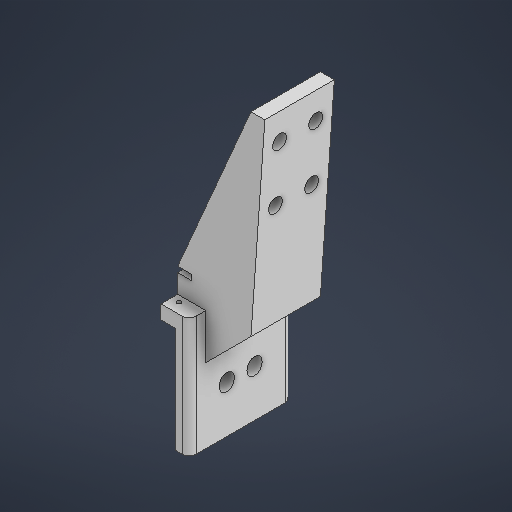
# Autodesk Inventor part: Camera_Bracket
Saved by Autodesk Inventor 2026 (Build 300175000, 175)
## iProperties
Created: 2025-04-19
Part Number: Camera_Bracket
Material: Generic
Document SubType Name: Modeling
Designer: Charl
Density: 1 g/cm^3
Appearance: Default
Author: Charl
Autodesk Inventor part; units mm, degrees
sketch "Sketch1" plane through (0, 0, 0) normal (0, 1, 0) x (-1, 0, 0)
  line L0 (-5.5, -37) -> (5.5, -37)
  line L1 (5.5, -37) -> (5.5, 37)
  line L2 (5.5, 37) -> (-5.5, 37)
  line L3 (-5.5, 37) -> (-5.5, -37)
  line L4 (-5.5, -37) -> (5.5, 37) construction
  line L5 (5.5, -37) -> (-5.5, 37) construction
  line L6 (-5.5, -25) -> (5.5, -25)
  line L7 (5.5, -25) -> (5.5, 25)
  line L8 (5.5, 25) -> (-5.5, 25)
  line L9 (-5.5, 25) -> (-5.5, -25)
  line L10 (-5.5, -25) -> (5.5, 25) construction
  line L11 (5.5, -25) -> (-5.5, 25) construction
  circle A0 centre (0, 29.5) radius 1.5
  circle A1 centre (0, -29.5) radius 1.5
  point P0 (0, 0)
  point P1 (0, -37)
  dimension "d0" = 74
  dimension "d1" = 11
  dimension "d2" = 11
  dimension "d3" = 50
  dimension "d4" = 3
  dimension "d5" = 7.5
  dimension "d6" = 3
  dimension "d7" = 7.5
  constraints: 24 end point, 5 midpoint, 4 parallel, 2 centre point, 2 horizontal, 2 perpendicular
  measures "d0" distance of L0.end L1.end
  measures "d1" distance of L1.end L2.end
  measures "d2" distance of L8.end L7.end
  measures "d3" distance of L7.end L6.end
  measures "d4" diameter of A0
  measures "d5" distance from line of A0.centre L2
  measures "d6" diameter of A1
  measures "d7" distance of point (0, -37) A1.centre
extrude "Extrusion1" add sketch "Sketch1" along normal blind 10
sketch "Sketch2" plane through (0, 10, 0) normal (0, 1, 0) x (1, 0, 0)
  line L0 (5.5, 37) -> (-5.5, 37) projected
  line L1 (4.8, 37) -> (14.8, 37)
  line L2 (14.8, 37) -> (14.8, -37)
  line L3 (14.8, -37) -> (4.8, -37)
  line L4 (4.8, -37) -> (4.8, 37)
  line L5 (5.5, -37) -> (5.5, 37) projected
  point P0 (0, 0)
  dimension "d10" = 74
  dimension "d11" = 0.7
  dimension "d12" = 10
  constraints: 8 end point, 2 parallel, 1 horizontal, 1 perpendicular, 1 point on line
  measures "d10" distance of L1.end L2.end
  measures "d11" distance between parallel lines of L5 L4
  measures "d12" distance of L1.start L1.end
extrude "Extrusion2" add sketch "Sketch2" against normal blind 86
ref_plane "Work Plane1" through (-5.5, 0, 0) normal (0, 0, 1) x (1, 0, 0)
sketch "Sketch3" plane through (-5.5, 0, 0) normal (0, 0, 1) x (1, 0, 0)
  line L0 (20.3, 10) -> (0, 10) projected
  line L1 (0, 10) -> (0, 27.494)
  line L2 (0, 27.494) -> (0.055, 27.494)
  line L3 (20.3, 10) -> (20.3, -76) projected
  line L4 (20.3, 10) -> (20.3, -22.405)
  line L5 (20.3, 10) -> (52.705, 10) construction
  line L6 (20.3, -22.405) -> (52.705, 10)
  line L7 (20.3, -22.405) -> (66.1276, -22.405) construction
  line L8 (52.705, 10) -> (52.705, 310)
  line L9 (52.705, 10) -> (352.705, 10) construction
  line L10 (0.055, 27.494) -> (10.055, 27.494) construction
  line L11 (52.705, 101.8003) -> (42.705, 101.8003) construction
  line L12 (42.705, 101.8003) -> (42.705, 219.1463) construction
  line L13 (42.705, 101.8003) -> (160.051, 101.8003) construction
  line L14 (0.055, 27.494) -> (42.705, 126.7645)
  line L15 (42.705, 126.7645) -> (52.705, 126.7645)
  point P0 (5.5, 0)
  dimension "d15" = 17.494
  dimension "d18" = 32.405
  dimension "d19" = 90
  dimension "d20" = 45
  dimension "d22" = 90
  dimension "d23" = 10
  dimension "d25" = 10
  dimension "d27" = 90
  dimension "d79" = 66.75
  constraints: 28 end point, 6 horizontal, 4 equal length, 3 point on line, 2 vertical, 1 collinear, 1 perpendicular
  measures "d15" distance of L0.end L1.end
  measures "d18" distance of L0.start L4.end
  measures "d19" angle of L4 L5
  measures "d20" angle of L7 L6
  measures "d22" angle of L9 L8
  measures "d23" distance of L2.end L10.end
  measures "d25" distance of L11.start L11.end
  measures "d27" angle of L13 L12
  measures "d79" angle of L10 L14
extrude "Extrusion3" add sketch "Sketch3" along normal mid plane 50
ref_plane "Work Plane2" through (-5.5, 27.494, 0) normal (-0.3947, -0.9188, 0) x (0, 0, 1)
sketch "Sketch4" plane through (-5.5, 0, 25) normal (0, 0, 1) x (1, 0, 0)
  line L0 (0, 0) -> (0, 10) construction
  line L1 (0, 10) -> (0, 23.494) construction
  line L2 (0, 23.494) -> (10, 23.494)
  line L3 (10, 23.494) -> (10, 27.494)
  line L4 (10, 27.494) -> (0, 27.494)
  line L5 (0, 27.494) -> (0, 23.494)
  point P0 (5.5, 0)
  dimension "d31" = 13.494
  dimension "d32" = 10
  dimension "d33" = 4
  constraints: 10 end point, 2 parallel, 1 horizontal, 1 perpendicular
  measures "d31" distance of L0.end L1.end
  measures "d32" distance of L4.end L3.end
  measures "d33" distance of L3.end L2.end
extrude "Extrusion4" cut sketch "Sketch4" against normal blind 269.75
sketch "Sketch5" plane through (-5.5, 27.494, 0) normal (-0.3947, -0.9188, 0) x (0, 0, 1)
  circle A0 centre (0, 14.9495) radius 25
  line L0 (-25, -0.0505) -> (25, -0.0505) projected
  point P0 (0, -15.9064)
  dimension "d36" = 50
  dimension "d37" = 15
  constraints: 1 centre point
  measures "d36" diameter of A0
  measures "d37" distance from line of L0 A0.centre
ref_plane "Work Plane3" through (37.205, 87.7645, 25) normal (0, 1, 0) x (1, 0, 0)
extrude "Extrusion5" cut sketch "Sketch5" along normal blind 54.3375 and the other way blind 67.371
ref_plane "Work Plane5" through (10.2593, -73.9067, 37) normal (-0.9081, 0.4187, 0) x (0, 0, 1)
ref_plane "Work Plane4" through (14.8, -76, 37) normal (-0.9081, 0.4187, 0) x (0, 0, 1)
sketch "Sketch6" plane through (10.2593, -73.9067, 37) normal (-0.9081, 0.4187, 0) x (0, 0, 1)
  line L0 (-74, 0) -> (0, 0) projected
  circle A0 centre (-37, 54.5) radius 5.5
  circle A1 centre (-37, 54.5) radius 2
  line L1 (-37, -200) -> (-37, 49)
  line L2 (-37, 60) -> (-37, 200)
  circle A2 centre (-47, 30.8) radius 5.5
  circle A3 centre (-47, 30.8) radius 2
  circle A4 centre (-27, 30.8) radius 5.5
  circle A5 centre (-27, 30.8) radius 2
  point P0 (-37, 62.8227)
  point P1 (-37, 0)
  dimension "d43" = 400
  dimension "d44" = 11
  dimension "d45" = 4
  dimension "d46" = 11
  dimension "d47" = 4
  dimension "d48" = 54.5
  dimension "d49" = 23.7
  dimension "d91" = 10
  constraints: 6 centre point, 4 end point, 3 coincident, 2 point on circle, 2 point on line, 2 symmetric about line, 2 vertical, 1 midpoint, 2 other
  measures "d43" distance of L1.start L2.end
  measures "d44" diameter of A0
  measures "d45" diameter of A1
  measures "d46" diameter of A2
  measures "d47" diameter of A3
  measures "d48" distance from line of L0 A0.centre
  measures "d49" vertical distance of A2.centre A0.centre
  measures "d91" distance from line of L1 A2.centre
extrude "Extrusion6" cut sketch "Sketch6" along normal blind 15 contours A0 | A1 | A2 | A3 | A4 | A5
extrude "Extrusion7" cut sketch "Sketch6" along normal blind 25.925 contours A0 | A1
extrude "Extrusion8" cut sketch "Sketch6" along normal blind 34.505 contours A1 | A3 | A5
ref_plane "Work Plane6" through (69.3627, 112.9485, -25) normal (-0.9188, 0.3947, 0) x (0, 0, 1)
sketch "Sketch7" plane through (69.3627, 112.9485, -25) normal (-0.9188, 0.3947, 0) x (0, 0, 1)
  line L0 (0, 0) -> (50, 0) projected
  line L1 (25, 150) -> (25, -150)
  line L2 (25, 150) -> (325, 150) construction
  line L3 (38, 10) -> (12, 10) construction
  line L4 (12, 10) -> (12, -29) construction
  line L5 (12, -29) -> (38, -29) construction
  line L6 (38, -29) -> (38, 10) construction
  circle A0 centre (38, 10) radius 2
  circle A1 centre (38, 10) radius 5
  circle A2 centre (38, -29) radius 2
  circle A3 centre (38, -29) radius 5
  circle A4 centre (12, 10) radius 2
  circle A5 centre (12, 10) radius 5
  circle A6 centre (12, -29) radius 2
  circle A7 centre (12, -29) radius 5
  line L7 (0, 3.9474) -> (50, 3.9474) projected
  point P0 (25, -131.1566)
  point P1 (25, 0)
  dimension "d57" = 300
  dimension "d58" = 90
  dimension "d63" = 26
  dimension "d64" = 39
  dimension "d67" = 4
  dimension "d68" = 10
  dimension "d69" = 10
  dimension "d70" = 4
  dimension "d78" = 13
  dimension "d85" = 10
  constraints: 12 end point, 8 centre point, 6 coincident, 4 symmetric about line, 2 horizontal, 2 midpoint, 2 parallel, 2 perpendicular, 1 vertical, 4 other
  measures "d57" distance of L1.start L1.end
  measures "d58" angle of L1 L2
  measures "d63" distance of L5.end L4.end
  measures "d64" distance of L4.end L3.end
  measures "d67" diameter of A0
  measures "d68" diameter of A1
  measures "d69" diameter of A3
  measures "d70" diameter of A2
  measures "d78" distance between parallel lines of L1 L6
  measures "d85" distance between parallel lines of L0 L3
fillet "Fillet1" radius 5 2 edges at (14.8, -33, 37) (14.8, -33, -37)
sketch "Sketch8" plane through (-5.5, 0, -25) normal (0, 0, -1) x (-1, 0, 0)
  line L0 (-52.705, 126.7645) -> (-42.705, 126.7645) construction
  line L1 (-42.705, 126.7645) -> (-52.705, 126.7645) construction
  line L2 (-52.705, 10) -> (-52.705, 126.7645) projected
  line L3 (-0.055, 27.494) -> (-42.705, 126.7645) projected
  line L4 (-42.705, 126.7645) -> (-52.705, 150.0402)
  line L5 (-52.705, 126.7645) -> (-42.705, 126.7645)
  line L6 (-52.705, 150.0402) -> (-62.705, 150.0402)
  line L7 (-62.705, 150.0402) -> (-52.705, 10)
  point P0 (-5.5, 0)
  dimension "d80" = 66.75
  dimension "d88" = 10
  constraints: 10 end point, 2 horizontal, 1 collinear, 1 point on line
  measures "d80" angle of L0 L4
  measures "d88" distance of L6.start L6.end
extrude "Extrusion13" add sketch "Sketch8" against normal blind 50
extrude "Extrusion9" cut sketch "Sketch7" along normal blind 28.9375 contours A0 | A1 | A2 | A3 | A4 | A5 | A6 | A7
extrude "Extrusion10" cut sketch "Sketch7" along normal blind 43.9375 contours A0 | A2 | A4 | A6
equation "\"d6\" = d4"
equation "\"d7\" = d5"
equation "\"d46\" = d44"
equation "\"d47\" = d45"
equation "\"d69\" = d68"
equation "\"d70\" = d67"
equation "\"d78\" = 0.5 * d63"
equation "\"d85\" = screw_offset"
equation "\"screw_offset\" = 10"
body "Solid1"
